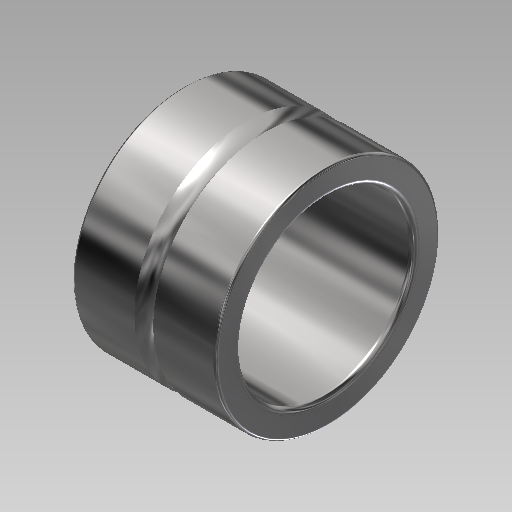
# Autodesk Inventor part: RF-1560ZZ_ir
Saved by Autodesk Inventor 2020 (Build 240168000, 168)
## iProperties
Created: 2019-10-06
Part Number: RF-1560ZZ_ir
Material: 鋼、炭素鋼
Catalog Web Link: www.cadenas.de
Description: Radial Flanged Ball Bearings (RF-Series/LF series) Metric ST ir-Radial Flanged Ball Bearings (RF-Series/LF series) Metric Shielded Type
Vendor: NMB
Document SubType Name: Modeling
Designer: psadmin
Manufacturer: NMB
Mass: 0.759069 g
Surface Area: 2.5052 cm^2
Volume: 0.0966967 cm^3
Density: 7.85 g/cm^3
Appearance: 半つや出し
Category: PARTsolutions
Company: NMB
PSOL_IDENT_0: {$CADENAS_DATA\23d-libs\nmb\pbbp\radial_flanged_ball_bearings\rfbb_rflfs_m\rflf_shielded_ir.prj},223
PSOL_IDENT_1: {VTYP=3D},{NB=RF-1560ZZ_ir},{LINA=RF-1560ZZ_ir},{NN=Radial Flanged Ball Bearings (RF-Series/LF seri
PSOL_IDENT_2: es) Metric ST ir},{DATE=11.11.2013 05:13:45},{GEOMDATE=24.10.2013 10:33:00},{VERSION=},{LINEID=1490}
PSOL_IDENT_3: ,{WBVAR=},{WBNUMERIC=}  {NB=RF-1560ZZ_ir},{LINA=RF-1560ZZ_ir},{KT=DUMMY},{IDNR=},{PN=RF-1560ZZ},{SHL
PSOL_IDENT_4: D=shielded},{FLANG=flanged},{SD=6.000},{D=15.000},{B=5.000},{SR=0.20},{BCZ=7},{DW=2.7781},{LI=7.80},
PSOL_IDENT_5: {LO=13.20},{D1=17.000},{C1=1.20},{D2=0.0},{C2=0.00},{COR=671},{CR=1058},{PCD=10.500},{U=13.278},{W=7
PSOL_IDENT_6: .722},{Y=1.389},{Z=1.389},{AA=13.000},{AC=1.00},{AD=0.000},{AF=0.00},{AQ=0.20},{AH=13.40},{AI=8.00},
PSOL_IDENT_7: {AJ=0.40}
NN: Radial Flanged Ball Bearings (RF-Series/LF series) Metric ST ir
NT: Radial Flanged Ball Bearings (RF-Series/LF series) Metric Shielded Type
NB: RF-1560ZZ_ir
NBSYN: $PN._ir
LINA: RF-1560ZZ_ir
PN: RF-1560ZZ
SHLD: shielded
FLANG: flanged
SD: 6
D: 15
B: 5
SR: 0.2
BCZ: 7
DW: 2.7781
LI: 7.8
LO: 13.2
D1: 0
C1: 1.2
D2: 0
C2: 0
COR: 671
CR: 1058
PCD: 10.5
U: 13.278
W: 7.722
Y: 1.389
Z: 1.389
AA: 13
AC: 1
AD: 0
AF: 0
AQ: 0.2
AH: 13.4
AI: 8
AJ: 0.4
SUPPLIER: NMB
ARTICLENO: RF-1560ZZ_ir
BOMINFO: RF-1560ZZ_ir
CREATOR: CADENAS GmbH
Title: RF-1560ZZ_ir
Author: Cadenas PARTsolutions
Comments: Radial Flanged Ball Bearings (RF-Series/LF series) Metric Shielded Type
Autodesk Inventor part; units mm, degrees
sketch "Sketch_5" plane through (0, 0, 0) normal (0, 0, 1) x (1, 0, 0)
  line L0 (5, 0) -> (0, 0)
  line L1 (0, 3.8) -> (0, 3.2)
  arc A0 (0, 3.2) -> (0.2, 3) centre (0.2, 3.2) ccw
  line L2 (0.2, 3) -> (4.8, 3)
  arc A1 (4.8, 3) -> (5, 3.2) centre (4.8, 3.2) ccw
  line L3 (5, 3.2) -> (5, 3.8)
  arc A2 (5, 3.8) -> (4.9, 3.9) centre (4.9, 3.8) ccw
  line L4 (4.9, 3.9) -> (2.827, 3.9)
  arc A3 (2.173, 3.9) -> (2.827, 3.9) centre (2.5, 5.25) ccw
  line L5 (2.173, 3.9) -> (0.1, 3.9)
  arc A4 (0.1, 3.9) -> (0, 3.8) centre (0.1, 3.8) ccw
  constraints: 12 end point, 10 point on circle, 5 centre point
revolve "Revolution1" add sketch "Sketch_5" angle 360 about axis through (5, 0, 0) along (1, 0, 0)
ref_plane "1_XY" through (2.5, 0, 0) normal (1, 0, 0) x (0, 0, -1)
ref_plane "1_YZ" through (2.5, 0, 0) normal (0, 0, -1) x (0, 1, 0)
ref_plane "1_ZX" through (2.5, 0, 0) normal (0, 1, 0) x (1, 0, 0)
ref_plane "Dummy_XY" through (0, 0, 0) normal (1, 0, 0) x (0, 0, -1)
ref_plane "Dummy_YZ" through (0, 0, 0) normal (0, 0, -1) x (0, 1, 0)
ref_plane "Dummy_ZX" through (0, 0, 0) normal (0, 1, 0) x (1, 0, 0)
ref_plane "shield1_XY" through (0.4, 0, 0) normal (1, 0, 0) x (0, 0, -1)
ref_plane "shield1_YZ" through (0.4, 0, 0) normal (0, 0, -1) x (0, 1, 0)
ref_plane "shield1_ZX" through (0.4, 0, 0) normal (0, 1, 0) x (1, 0, 0)
ref_plane "shield2_XY" through (4.6, 0, 0) normal (-1, 0, 0) x (0, 0, -1)
ref_plane "shield2_YZ" through (4.6, 0, 0) normal (0, 0, -1) x (0, -1, 0)
ref_plane "shield2_ZX" through (4.6, 0, 0) normal (0, -1, 0) x (-1, 0, 0)
body "Solid1"
